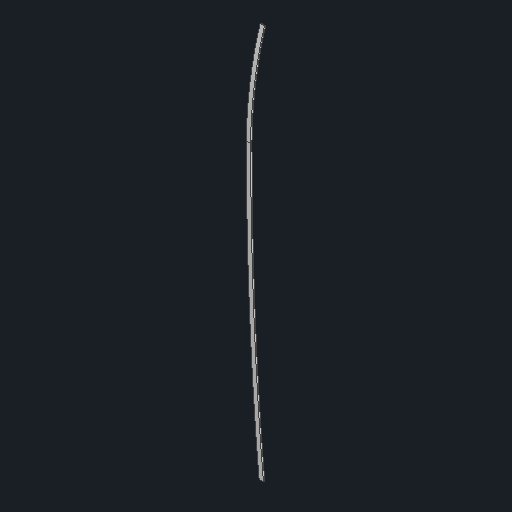
# Autodesk Inventor part: sealing_liner
Saved by Autodesk Inventor 2024 (Build 280153000, 153)
## iProperties
Created: 2022-03-25
Part Number: sealing_liner
Material: Generic
Document SubType Name: Modeling
Designer: kardo
Density: 1 g/cm^3
Appearance: Default
Mass: 3.41892 g
Surface Area: 59.4112 cm^2
Volume: 3.41892 cm^3
Author: kardo
Autodesk Inventor part; units mm, degrees
ref_plane "YZ Plane" through (0, 0, 0) normal (1, 0, 0) x (0, 1, 0)
ref_plane "XZ Plane" through (0, 0, 0) normal (0, 1, 0) x (-1, 0, 0)
ref_plane "XY Plane" through (0, 0, 0) normal (0, 0, 1) x (1, 0, 0)
derived "parameters_frame.ipt"
derived "surface_body.ipt"
sketch "sk_rail_top_symmetry" plane through (0, 0, 0) normal (1, 0, 0) x (0, 1, 0)
  line L0 (0, 107.6209) -> (0, -224.5198) construction
  line L1 (0, 54.4) -> (-345, 54.4) construction
  line L2 (-345, 107.6209) -> (-345, -224.5198) construction
  line L3 (112.2, 107.6209) -> (112.2, -224.5198) construction
  line L4 (0, 54.4) -> (37.026, 54.4) construction
  line L5 (37.026, 54.4) -> (80.784, 47.9917) construction
  line L6 (80.784, 47.9917) -> (112.2, 37.536) construction
  line L7 (-469.3291, 0) -> (375.7215, 0) construction
  spline S0 degree 2 poles (-345, 39.712) (-172.656, 54.3934) (0, 54.4) knots 0 0 0 1 1 1
  spline S1 degree 3 poles (0, 54.4) (37.026, 54.4) (80.784, 47.9917) (112.2, 37.536) knots 1 1 1 1 2 2 2 2
  point P0 (0, 0)
  point P1 (-172.5, 50.728)
  point P2 (112.2, 28.832)
ref_plane "plane_symmetry" through (0, 0, 0) normal (1, 0, 0) x (0, 1, 0)
sketch "sk_base" plane through (0, 0, 0) normal (1, 0, 0) x (0, 1, 0)
  spline S0 degree 2 poles (-345, 39.712) (-172.656, 54.3934) (0, 54.4) knots 0 0 0 1 1 1 projected
  spline S1 degree 3 poles (0, 54.4) (37.026, 54.4) (80.784, 47.9917) (112.2, 37.536) knots 1 1 1 1 2 2 2 2 projected
  line L0 (-344.8727, 38.2174) -> (-345, 39.712)
  line L1 (109.2, 38.5104) -> (108.7467, 37.0805)
  spline S2 degree 4 poles (-344.8727, 38.2174) (-258.862, 45.5443) (-172.6445, 50.447) (-86.3222, 52.8967) (0.0001, 52.9) knots 0 0 0 0 0 1 1 1 1 1
  spline S3 degree 5 poles (0, 52.9) (11.6418, 52.8997) (23.2822, 52.3712) (34.8945, 51.44) (56.8204, 48.9455) (78.5329, 45.0107) (88.7161, 42.8071) (98.8205, 40.2269) (108.7467, 37.0803) knots 0 0 0 0 0 0 0.527853 0.527853 0.527853 1 1 1 1 1 1
  point P0 (0, 0)
  dimension "d7" = 1.5
  dimension "d8" = 3
  constraints: 4 end point, 9 other
  measures "d8" horizontal distance of point (112.2, 37.536) L1.start
extrude "thicken" add sketch "sk_base" along normal blind 5
equation "\"d7\" = cowl_liner_thickness"
equation "\"d8\" = bulkhead_thickness"
equation "\"d9\" = cowl_sealing_width"
equation "\"cowl_liner_thickness\" = 1.5"
equation "\"cowl_sealing_width\" = 5"
equation "\"bulkhead_thickness\" = 3"
body "Solid2"
